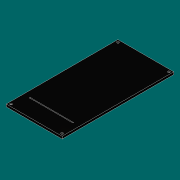
# Autodesk Inventor part: topBottom
Saved by Autodesk Inventor 2016 SP1 (Build 200210100, 210)
## iProperties
Created: 2015-10-13
Part Number: topBottom
Material: PC/ABS Plastic
Document SubType Name: Modeling
Designer: Sawaiz
Density: 0.357273 g/cm^3
Appearance: Smooth - Black
Author: Sawaiz
Autodesk Inventor part; units mm, degrees
ref_plane "YZ Plane" through (0, 0, 0) normal (1, 0, 0) x (0, 1, 0)
ref_plane "XZ Plane" through (0, 0, 0) normal (0, 1, 0) x (-1, 0, 0)
ref_plane "XY Plane" through (0, 0, 0) normal (0, 0, 1) x (1, 0, 0)
sketch "Sketch1" plane through (0, 0, 0) normal (0, 0, 1) x (1, 0, 0)
  line L0 (-146.05, -73.025) -> (146.05, -73.025)
  line L1 (146.05, -73.025) -> (146.05, 73.025)
  line L2 (146.05, 73.025) -> (-146.05, 73.025)
  line L3 (-146.05, 73.025) -> (-146.05, -73.025)
  line L4 (-146.05, -73.025) -> (146.05, 73.025) construction
  line L5 (146.05, -73.025) -> (-146.05, 73.025) construction
  point P0 (0, 0)
  dimension "d0" = 292.1
  dimension "d1" = 146.05
  constraints: 12 end point, 2 midpoint, 2 parallel, 1 horizontal, 1 perpendicular
  measures "d0" distance of L2.end L1.end
  measures "d1" distance of L1.end L0.end
extrude "Extrusion1" add sketch "Sketch1" along normal blind 9.525
sketch "Sketch12" plane through (0, 0, 9.525) normal (0, 0, 1) x (1, 0, 0)
  line L0 (-146.05, -73.025) -> (146.05, -73.025) projected
  line L1 (146.05, -73.025) -> (146.05, 73.025) projected
  line L2 (146.05, 73.025) -> (-146.05, 73.025) projected
  line L3 (-146.05, 73.025) -> (-146.05, -73.025) projected
  line L4 (139.7, -66.675) -> (-139.7, -66.675)
  line L5 (-139.7, -66.675) -> (-139.7, 66.675)
  line L6 (-139.7, 66.675) -> (139.7, 66.675)
  line L7 (139.7, 66.675) -> (139.7, -66.675)
  point P0 (0, 0)
  dimension "d87" = 6.35
  constraints: 8 end point, 4 coincident, 3 other
  measures "d87" distance between parallel lines of L0 L4
hole "Hole6" at (139.7, -66.675, 9.525) at (-139.7, -66.675, 9.525) at (-139.7, 66.675, 9.525) at (139.7, 66.675, 9.525) direction (0, 0, -1) diameter 3.264 end through all countersink diameter 5.715 countersink angle 82 clearance for "Flat Head Machine Screw (82)" size "#4" standard "Ansi Unified Screw Threads"
sketch "Sketch13" plane through (0, 0, 0) normal (0, 0, -1) x (-1, 0, 0)
  circle A0 centre (139.7, 66.675) radius 1.632 projected
  circle A1 centre (-139.7, -66.675) radius 1.632 projected
  circle A2 centre (139.7, -66.675) radius 1.632 projected
  circle A3 centre (-139.7, 66.675) radius 1.632 projected
  line L0 (146.05, -73.025) -> (-146.05, -73.025) projected
  line L1 (146.05, 73.025) -> (146.05, -73.025) projected
  line L2 (-146.05, 73.025) -> (146.05, 73.025) projected
  line L3 (-146.05, -73.025) -> (-146.05, 73.025) projected
  line L4 (-136.525, 63.5) -> (136.525, 63.5)
  line L5 (136.525, 63.5) -> (136.525, -63.5)
  line L6 (136.525, -63.5) -> (-136.525, -63.5)
  line L7 (-136.525, -63.5) -> (-136.525, 63.5)
  point P0 (0, 0)
  dimension "d95" = 9.525
  constraints: 8 end point, 3 other
  measures "d95" distance between parallel lines of L3 L7
extrude "Extrusion6" cut sketch "Sketch13" against normal blind 3.175
sketch "Sketch14" plane through (0, 0, 3.175) normal (0, 0, -1) x (-1, 0, 0)
  line L0 (-136.525, 63.5) -> (-136.525, -63.5) projected
  line L1 (136.525, 63.5) -> (-136.525, 63.5) projected
  line L2 (136.525, -63.5) -> (136.525, 63.5) projected
  line L3 (-136.525, -63.5) -> (136.525, -63.5) projected
  circle A0 centre (-139.7, 66.675) radius 1.632 projected
  circle A1 centre (139.7, -66.675) radius 1.632 projected
  circle A2 centre (-139.7, -66.675) radius 1.632 projected
  circle A3 centre (139.7, 66.675) radius 1.632 projected
  line L4 (146.05, -73.025) -> (-146.05, -73.025) projected
  line L5 (146.05, 73.025) -> (146.05, -73.025) projected
  line L6 (-146.05, 73.025) -> (146.05, 73.025) projected
  line L7 (-146.05, -73.025) -> (-146.05, 73.025) projected
  line L8 (-136.525, 63.5) -> (-136.525, -63.5) projected
  line L9 (-136.525, -63.5) -> (136.525, -63.5) projected
  line L10 (136.525, -63.5) -> (136.525, 63.5) projected
  line L11 (136.525, 63.5) -> (-136.525, 63.5) projected
  line L12 (-140.0429, 71.4375) -> (140.0429, 71.4375)
  line L13 (144.4625, 67.0179) -> (144.4625, -67.0179)
  line L14 (140.0429, -71.4375) -> (-140.0429, -71.4375)
  line L15 (-144.4625, -67.0179) -> (-144.4625, 67.0179)
  line L16 (-140.0429, 69.2277) -> (140.0429, 69.2277)
  line L17 (142.2527, 67.0179) -> (142.2527, -67.0179)
  line L18 (140.0429, -69.2277) -> (-140.0429, -69.2277)
  line L19 (-142.2527, -67.0179) -> (-142.2527, 67.0179)
  arc A4 (-142.2527, -67.0179) -> (-140.0429, -69.2277) centre (-140.0429, -67.0179) ccw
  arc A5 (-140.0429, 69.2277) -> (-142.2527, 67.0179) centre (-140.0429, 67.0179) ccw
  arc A6 (142.2527, 67.0179) -> (140.0429, 69.2277) centre (140.0429, 67.0179) ccw
  arc A7 (140.0429, -69.2277) -> (142.2527, -67.0179) centre (140.0429, -67.0179) ccw
  arc A8 (-144.4625, -67.0179) -> (-140.0429, -71.4375) centre (-140.0429, -67.0179) ccw
  arc A9 (-140.0429, 71.4375) -> (-144.4625, 67.0179) centre (-140.0429, 67.0179) ccw
  arc A10 (144.4625, 67.0179) -> (140.0429, 71.4375) centre (140.0429, 67.0179) ccw
  arc A11 (140.0429, -71.4375) -> (144.4625, -67.0179) centre (140.0429, -67.0179) ccw
  point P0 (0, 0)
  dimension "d101" = 1.5875
  dimension "d102" = 3.7973
  dimension "d103" = 2.2098
  dimension "d104" = 4.4196
  constraints: 16 end point, 16 point on circle, 16 tangent, 8 centre point, 6 equal radius, 6 other
  measures "d101" distance between parallel lines of L7 L15
  measures "d102" distance between parallel lines of L7 L19
  measures "d103" radius of A4
  measures "d104" radius of A8
extrude "Extrusion7" cut sketch "Sketch14" against normal blind 1.1684 contours L12 A10 L13 A11 L14 A8 L15 A9
sketch "Sketch15" plane through (0, 0, 9.525) normal (0, 0, 1) x (1, 0, 0)
  circle A0 centre (-139.7, 66.675) radius 2.8575 projected
  circle A1 centre (139.7, -66.675) radius 2.8575 projected
  circle A2 centre (-139.7, -66.675) radius 2.8575 projected
  circle A3 centre (139.7, 66.675) radius 2.8575 projected
  line L0 (-146.05, -73.025) -> (146.05, -73.025) projected
  line L1 (146.05, -73.025) -> (146.05, 73.025) projected
  line L2 (146.05, 73.025) -> (-146.05, 73.025) projected
  line L3 (-146.05, 73.025) -> (-146.05, -73.025) projected
  line L4 (101.799, -57.15) -> (99.799, -57.15)
  line L5 (99.799, -57.15) -> (99.799, 57.15)
  line L6 (99.799, 57.15) -> (101.799, 57.15)
  line L7 (101.799, 57.15) -> (101.799, -57.15)
  point P0 (0, 0)
  dimension "d107" = 2
  dimension "d108" = 44.251
  dimension "d109" = 15.875
  dimension "d110" = 15.875
  constraints: 8 end point, 2 parallel, 1 horizontal, 1 perpendicular
  measures "d107" distance of L4.start L4.end
  measures "d108" distance between parallel lines of L1 L7
  measures "d109" distance between parallel lines of L0 L4
  measures "d110" distance between parallel lines of L2 L6
extrude "Extrusion8" cut sketch "Sketch15" against normal through all contours L4 L5 L6 L7
fillet "Fillet2" radius 1 4 edges at (99.799, 57.15, 4.7625) (101.799, 57.15, 4.7625) (99.799, -57.15, 4.7625) (101.799, -57.15, 4.7625)
equation "\"d0\" = depth + 2 * frameAcrylicThickness"
equation "\"d1\" = width + 2 * frameAcrylicThickness"
equation "\"d2\" = frameAcrylicThickness"
equation "\"d95\" = frameAcrylicThickness"
equation "\"d108\" = -centerThickness + aerogelThickness + frameAcrylicThickness + internalAcrylicThickness - fresnelThickness"
equation "\"d109\" = frameAcrylicThickness + internalAcrylicThickness"
equation "\"d110\" = frameAcrylicThickness + internalAcrylicThickness"
equation "\"acrylicThickness\" = 9.525"
equation "\"width\" = 127"
equation "\"depth\" = 273.05"
equation "\"aerogelThickness\" = 30"
equation "\"oRingWidth\" = 1.5875"
equation "\"mirrorGroove\" = 19.05"
equation "\"mirrorGrooveMill\" = 3.175"
equation "\"height\" = 127"
equation "\"mirrorAngle\" = 5deg"
equation "\"detectorWidth\" = 52"
equation "\"detectorHeight\" = 52"
equation "\"mirrorThickness\" = 3.175"
equation "\"fresnelThickness\" = 0.1"
equation "\"focalLength\" = 76.2"
equation "\"ior\" = 1.49"
equation "\"centerThickness\" = 1.524"
equation "\"fresnelAngle\" = 90deg"
equation "\"fresnelEffectiveDiameter\" = 152.4"
equation "\"mirrorSuppourtWidth\" = 38.1"
equation "\"backGrooveBit\" = 4.8006"
equation "\"sensorHolderWidth\" = 88.9"
equation "\"sensorHolderHeight\" = 88.9"
equation "\"sensorHolderSensorHeight\" = 53.975"
equation "\"sensorHolderSensorWidth\" = 53.975"
equation "\"sensorHolderORingID\" = 203.2"
equation "\"sensorHolderFlushORingID\" = 304.8"
equation "\"frontBackORingID\" = 419.1"
equation "\"backMirrorGroove\" = 6.35"
equation "\"fresnelChamfer\" = 6.35"
equation "\"fresnelMirrorChamfer\" = 6.35"
equation "\"detectorOpeningHeight\" = 76.2"
equation "\"detectorOpeningWidth\" = 76.2"
equation "\"sensorHolderDepth\" = 19.05"
equation "\"frameAcrylicThickness\" = 9.525"
equation "\"internalAcrylicThicnkess\" = 6.35"
equation "\"internalAcrylicThickness\" = 6.35"
equation "\"aerogelClearence\" = 3.175"
equation "\"backplanePCBWidth\" = 76.2"
equation "\"backplaneHoleOffsett\" = 6.35"
equation "\"backplanePCBHeight\" = 76.2"
equation "\"backplanePostionOffsett\" = 12.7"
equation "\"moduleSlotClearence\" = 0.79375"
body "Solid1"
